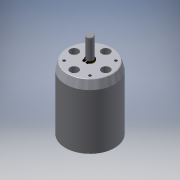
# Autodesk Inventor part: Turnigy Brushless DC Motor
Saved by Autodesk Inventor 2018 (Build 220112000, 112)
## iProperties
Created: 2018-02-13
Part Number: Turnigy Brushless DC Motor
Material: Generic
Document SubType Name: Modeling
Designer: ruben
Density: 1 g/cm^3
Sheet Metal Rule: Default_mm
Appearance: Default
Mass: 200.69 g
Surface Area: 274.821 cm^2
Volume: 200.69 cm^3
Author: ruben
Autodesk Inventor part; units mm, degrees
ref_plane "YZ Plane" through (0, 0, 0) normal (1, 0, 0) x (0, 1, 0)
ref_plane "XZ Plane" through (0, 0, 0) normal (0, 1, 0) x (-1, 0, 0)
ref_plane "XY Plane" through (0, 0, 0) normal (0, 0, 1) x (1, 0, 0)
sketch "Sketch3" plane through (0, 0, 0) normal (0, 0, 1) x (1, 0, 0)
  line L0 (-41.3, 0) -> (41.3, 0) projected
  line L1 (0, -41.3) -> (0, 41.3) projected
  circle A0 centre (0, 0) radius 29.5
  circle A1 centre (0, 0) radius 4
  circle A2 centre (0, 0) radius 8.25
  dimension "d0" = 59
  dimension "d1" = 8
  dimension "d4" = 16.5
  constraints: 3 centre point, 3 coincident
  measures "d0" diameter of A0
  measures "d1" diameter of A1
  measures "d4" diameter of A2
extrude "Extrusion1" add sketch "Sketch3" along normal blind 84.3 contours A1 L1 A2 L0 | L0 A2 L1 A1 | A2 L1 A0 L0 | L0 A0 L1 A2 | A1 L0 A2 L1 | L1 A2 L0 A1 | A2 L0 A0 L1 | L1 A0 L0 A2
extrude "Extrusion2" add sketch "Sketch3" against normal blind 2 contours A1 L1 A2 L0 | L0 A2 L1 A1 | A1 L0 A2 L1 | L1 A2 L0 A1
sketch "Sketch4" plane through (0, 0, 84.3) normal (0, 0, 1) x (1, 0, 0)
  line L0 (-17.5962, -17.5962) -> (17.2802, 17.2802) construction
  line L1 (0, -41.3) -> (0, 41.3) projected
  circle A0 centre (0, 0) radius 22 construction
  circle A1 centre (0, 0) radius 27
  circle A2 centre (0, 0) radius 8.25 projected
  circle A3 centre (0, 0) radius 19 construction
  line L2 (-41.3, 0) -> (41.3, 0) projected
  point P0 (-15.5563, -15.5563)
  point P1 (-19, 0)
  dimension "d8" = 44
  dimension "d26" = 38
  dimension "d7" = 45
  dimension "d19" = 54
  constraints: 3 coincident, 3 point on line, 2 end point, 1 centre point, 1 horizontal alignment, 5 other
  measures "d7" angle of L1 L0
  measures "d19" diameter of A1
hole "Hole1" at (-15.5563, -15.5563, 84.3) direction (0, 0, -1) diameter 3.242 depth 10 thread size "M4x0.7" class "6H" standard "ISO Metric profile"
pattern_circular "Circular Pattern1" count 4 over 360 about axis through (0, 0, -10) along (0, 0, 1) of "Hole1"
chamfer "Chamfer1" distance 2.5 distance2 10 1 edges at (-29.5, 0, 84.3) measured on face at (16.4172, -4.6491, 84.3)
chamfer "Chamfer2" distance 0.5 angle 45 1 edges at (-27, 0, 84.3)
hole "Hole2" at (-19, 0, 84.3) direction (0, 0, -1) diameter 10 depth 10
pattern_circular "Circular Pattern2" count 4 over 360 about axis through (0, 0, -10) along (0, 0, 1) of "Hole2"
sketch "Sketch5" plane through (0, 0, 0) normal (0, 0, -1) x (-1, 0, 0)
  circle A0 centre (0, 0) radius 5
  dimension "d37" = 10
  constraints: 1 centre point, 1 coincident
  measures "d37" diameter of A0
extrude "Extrusion3" add sketch "Sketch5" along normal blind 3.5
sketch "Sketch6" plane through (0, 0, 0) normal (0, 0, 1) x (1, 0, 0)
  circle A0 centre (0, 0) radius 4
  dimension "d40" = 8
  constraints: 1 centre point, 1 coincident
  measures "d40" diameter of A0
extrude "Extrusion4" add sketch "Sketch6" along normal blind 110.8
chamfer "Chamfer3" distance 0.5 angle 45 1 edges at (-4, 0, 110.8)
sketch "Sketch7" plane through (0, 0, 0) normal (0, 0, -1) x (-1, 0, 0)
  circle A0 centre (0, 0) radius 15 construction
  dimension "d46" = 30
  constraints: 1 centre point, 1 coincident
  measures "d46" diameter of A0
chamfer "Chamfer4" distance 14.5 distance2 8 1 edges at (-29.5, 0, 0) measured on face at (22.051, -3.0114, 0)
fillet "Fillet1" radius 1.5 1 edges at (-15, 0, 0)
sketch "Sketch8" plane through (0, 0, 0) normal (0, 0, -1) x (-1, 0, 0)
  line L0 (15.8398, 15.8398) -> (-19.5223, -19.5223) construction
  line L1 (0, -41.3) -> (0, 41.3) projected
  circle A0 centre (0, 0) radius 10 construction
  point P0 (7.0711, 7.0711)
  dimension "d52" = 20
  dimension "d51" = 45
  constraints: 2 end point, 2 point on line, 1 coincident, 3 other
  measures "d51" angle of L1 L0
hole "Hole3" at (-7.0711, 7.0711, 0) direction (0, 0, 1) diameter 3.242 depth 11.8 thread size "M4x0.7" class "6H" standard "ISO Metric profile"
pattern_circular "Circular Pattern3" count 4 over 360 about axis through (0, 0, -10) along (0, 0, 1) of "Hole3"
sketch "Sketch9" plane through (0, 0, 0) normal (0, 0, -1) x (-1, 0, 0)
  line L0 (0, -41.3) -> (0, 41.3) projected
  line L1 (41.3, 0) -> (-41.3, 0) projected
  circle A0 centre (0, 0) radius 29.5 construction
  line L2 (13.9931, 4.9577) -> (22.4931, 7.1847)
  line L3 (13.9931, -4.9577) -> (22.4931, -7.1847)
  arc A1 (12.5421, -2.6148) -> (12.5421, 2.6148) centre (0, 0) ccw
  arc A2 (-25.4435, 5.3745) -> (-26.0049, 0) centre (0, 0) ccw
  arc A3 (24.9498, -5.6951) -> (24.9498, 5.6951) centre (0, 0) ccw
  arc A4 (24.9498, 5.6951) -> (22.4931, 7.1847) centre (23, 5.25) ccw
  arc A5 (22.4931, -7.1847) -> (24.9498, -5.6951) centre (23, -5.25) ccw
  arc A6 (12.5421, -2.6148) -> (13.9931, -4.9577) centre (14.5, -3.023) ccw
  arc A7 (13.9931, 4.9577) -> (12.5421, 2.6148) centre (14.5, 3.023) ccw
  line L4 (23, 25.8019) -> (23, -28.6173) construction
  point P0 (24.4098, 7.6869)
  point P1 (12.0177, 4.4402)
  point P2 (12.0177, -4.4402)
  point P3 (24.4098, -7.6869)
  dimension "d69" = 2
  dimension "d70" = 8.5
  dimension "d71" = 10.5
  dimension "d72" = 8.5
  dimension "d73" = 8.8804
  dimension "d74" = 23
  constraints: 18 point on circle, 8 point on line, 8 tangent, 7 centre point, 6 end point, 3 equal radius, 2 coincident, 1 parallel
  measures "d69" radius of A4
  measures "d70" horizontal distance of A7.centre A4.centre
  measures "d71" distance of A4.centre A5.centre
  measures "d72" horizontal distance of A6.centre A5.centre
  measures "d73" distance of point (12.018, 4.44) point (12.018, -4.44)
  measures "d74" distance between parallel lines of L0 L4
extrude "Extrusion5" cut sketch "Sketch9" against normal blind 10
pattern_circular "Circular Pattern4" count 5 over 360 about axis through (0, 0, -10) along (0, 0, 1) of "Extrusion5"
sketch "Sketch10" plane through (0, 0, 84.3) normal (0, 0, 1) x (1, 0, 0)
  circle A0 centre (0, 0) radius 5
  circle A1 centre (0, 0) radius 4
  dimension "d81" = 10
  dimension "d82" = 8
  constraints: 2 centre point, 2 coincident
  measures "d81" diameter of A0
  measures "d82" diameter of A1
extrude "Extrusion6" add sketch "Sketch10" along normal blind 1
sketch "Sketch11" plane through (0, 0, 85.3) normal (0, 0, 1) x (1, 0, 0)
  circle A0 centre (0, 0) radius 4
  arc A1 (3.5858, 3.5559) -> (3.5858, -3.5559) centre (0, 0) ccw
  circle A2 centre (0, 0) radius 4 projected
  line L0 (0, -41.3) -> (0, 41.3) projected
  line L1 (-41.3, 0) -> (41.3, 0) projected
  line L2 (3.8413, -1.1156) -> (6.1546, -1.1152)
  line L3 (3.8416, 1.1146) -> (6.1546, 1.1152)
  line L4 (6.1546, 1.1152) -> (6.1546, 3.1152)
  line L5 (6.1546, 1.1152) -> (8.1546, 1.1152) construction
  line L6 (6.1546, -1.1152) -> (6.1546, -3.1152)
  line L7 (6.1546, -1.1152) -> (8.1546, -1.1152) construction
  line L8 (6.1546, 3.1152) -> (3.5858, 3.5559)
  line L9 (6.1546, -3.1152) -> (3.5858, -3.5559)
  circle A3 centre (5.0046, -2.1152) radius 0.5
  circle A4 centre (5.0046, 2.1152) radius 0.5
  dimension "d85" = 8
  dimension "d86" = 10.1
  dimension "d91" = 2
  dimension "d92" = 90
  dimension "d94" = 2
  dimension "d95" = 90
  dimension "d98" = 3.1152
  dimension "d99" = 3.1152
  dimension "d100" = 2.3133
  dimension "d101" = 2.3131
  dimension "d102" = 3.5858
  dimension "d103" = 3.5858
  dimension "d104" = 1.1156
  dimension "d105" = 1.1146
  dimension "d106" = 1.15
  dimension "d107" = 1.0003
  dimension "d108" = 0.9998
  dimension "d109" = 1.15
  dimension "d110" = 1
  dimension "d111" = 1
  constraints: 16 end point, 4 coincident, 3 centre point, 3 point on circle, 2 horizontal, 2 perpendicular, 2 vertical, 3 other
  measures "d86" diameter of A1
  measures "d91" distance of L3.end L4.end
  measures "d92" angle of L5 L4
  measures "d94" distance of L2.end L6.end
  measures "d95" angle of L6 L7
  measures "d98" distance from line of L1 L6.end
  measures "d99" distance from line of L1 L4.end
  measures "d100" distance of L2.start L2.end
  measures "d101" distance of L3.start L3.end
  measures "d102" distance from line of L8.end L0
  measures "d103" distance from line of L9.end L0
  measures "d104" distance from line of L1 L2.start
  measures "d105" distance from line of L1 L3.start
  measures "d106" distance from line of L4 point (5.005, 2.115)
  measures "d107" distance from line of L3 point (5.005, 2.115)
  measures "d108" distance from line of L2 point (5.005, -2.115)
  measures "d109" distance from line of L6 point (5.005, -2.115)
  measures "d110" diameter of A3
  measures "d111" diameter of A4
extrude "Extrusion7" add sketch "Sketch11" along normal blind 1 contours A0 L0 A1 L8 L4 L3 | L2 L6 L9 A1 L0 A0 | A0 L1 A1 L0 | L0 A1 L1 A0
sketch "Sketch12" plane through (0, 0, 10) normal (0, 0, -1) x (-0.809017, -0.5877853, 0)
  circle A0 centre (0, 0) radius 26.5
  dimension "d114" = 53
  constraints: 1 centre point, 1 coincident
  measures "d114" diameter of A0
extrude "Extrusion8" cut sketch "Sketch12" against normal blind 5
equation "\"BendRadius\" = Thickness"
equation "\"BendReliefWidth\" = Thickness"
equation "\"BendReliefDepth\" = 0.5 * Thickness"
equation "\"CornerReliefSize\" = 4 * Thickness"
equation "\"MinimumRemnant\" = 2 * Thickness"
equation "\"TransitionRadius\" = BendRadius"
equation "\"JacobiRadiusSize\" = BendRadius"
equation "\"GapSize\" = Thickness"
equation "\"Thickness\" = 0.5"
body "Solid1"
